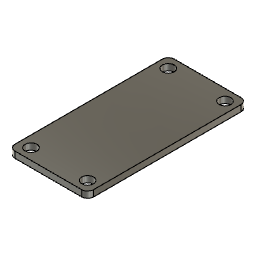
BT-Modul_BK3231 (Autodesk Fusion 360 design; units mm, degrees)
Autodesk Fusion 360 part; units mm, degrees
sketch "Sketch1" plane through (0, 0, 0) normal (0, 0, 1) x (1, 0, 0)
  line L0 (0, 0) -> (20, 0)
  line L1 (20, 0) -> (20, 40.5)
  line L2 (20, 40.5) -> (0, 40.5)
  line L3 (0, 40.5) -> (0, 0)
  line L4 (10, 40.5) -> (10, 0) construction
  circle A0 centre (2.8, 37.7) radius 1.5
  circle A1 centre (2.8, 2.8) radius 1.5
  circle A2 centre (17.2, 37.7) radius 1.5
  circle A3 centre (17.2, 2.8) radius 1.5
  dimension "d1" = 20
  dimension "d2" = 40.5
  dimension "d3" = 3
  dimension "d4" = 3
  dimension "d5" = 2.8
  dimension "d6" = 2.8
  dimension "d7" = 2.8
  dimension "d8" = 2.8
  constraint horizontal L0
  constraint vertical L1
  constraint horizontal L2
  constraint vertical L3
  constraint coincident L0.start L3.end
  constraint midpoint L2 L4.start
  constraint midpoint L0 L4.end
  constraint symmetric L4 A0 A2
  constraint symmetric L4 A1 A3
  measures "d1" distance of L0.start L0.end
  measures "d2" distance of L0.start L2.end
  measures "d3" diameter of A0
  measures "d4" diameter of A1
  measures "d5" distance of L3 A1.centre
  measures "d6" distance of L0 A1.centre
  measures "d7" distance of L3 A0.centre
  measures "d8" distance of L2 A0.centre
extrude "Extrude1" add sketch "Sketch1" along normal blind 1.6
fillet "Fillet1" radius 1.5 4 edges at (20, 0, 0.8) (20, 40.5, 0.8) (0, 40.5, 0.8) (0, 0, 0.8)
